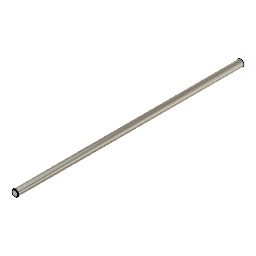
Linear_rail_Z_F01 (Autodesk Fusion 360 design; units mm, degrees)
Autodesk Fusion 360 part; units mm, degrees
cylinder "円柱プリミティブ1" add diameter 12 height 400 placed x (1, 0, 0) y (0, 0, -1) z (0, 1, 0) at (0, 0, 0)
chamfer "面取り1" distance 1 angle 45 2 edges at (-5.594, 400, 2.1697) (-5.594, 0, -2.1697)
